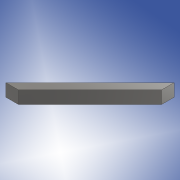
# Autodesk Inventor part: C002
Saved by Autodesk Inventor 2017 (Build 210142000, 142)
## iProperties
Created: 2017-06-13
Part Number: C002
Material: Steel, Carbon
Document SubType Name: Modeling
Designer: zallen
Density: 7.85 g/cm^3
Appearance: Semi-Polished
Mass: 163.378 g
Surface Area: 71.4944 cm^2
Volume: 20.8125 cm^3
Author: zallen
Autodesk Inventor part; units mm, degrees
ref_plane "YZ Plane" through (0, 0, 0) normal (1, 0, 0) x (0, 1, 0)
ref_plane "XZ Plane" through (0, 0, 0) normal (0, 1, 0) x (-1, 0, 0)
ref_plane "XY Plane" through (0, 0, 0) normal (0, 0, 1) x (1, 0, 0)
sketch "Sketch1" plane through (0, 0, 0) normal (0, 0, 1) x (1, 0, 0)
  line L0 (0, 0) -> (100, 0) construction
  line L1 (100, 0) -> (100, 100) construction
  line L2 (100, 100) -> (0, 100) construction
  line L3 (0, 100) -> (0, 0) construction
  line L4 (0, 0) -> (100, 100)
  line L5 (0, 0) -> (15, 0)
  line L6 (100, 100) -> (100, 85)
  line L7 (15, 0) -> (100, 85)
  dimension "d1" = 100
  dimension "d2" = 100
  dimension "d3" = 15
  dimension "d4" = 15
  constraints: 16 end point, 2 parallel, 2 point on line, 1 horizontal, 1 perpendicular
  measures "d1" distance of L2.end L1.end
  measures "d2" distance of L1.end L0.end
  measures "d3" distance of L0.start L5.end
  measures "d4" distance of L1.end L6.end
extrude "Extrusion1" add sketch "Sketch1" along normal blind 15
body "Solid1"
